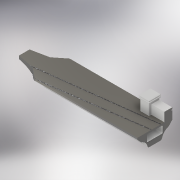
# Autodesk Inventor part: AC
Saved by Autodesk Inventor 2019 (Build 230136000, 136)
## iProperties
Created: 2020-08-10
Part Number: AC
Material: Generic
Document SubType Name: Modeling
Designer: Manoj
Density: 1 g/cm^3
Appearance: Default
Author: Manoj
Autodesk Inventor part; units mm, degrees
ref_plane "YZ Plane" through (0, 0, 0) normal (1, 0, 0) x (0, 1, 0)
ref_plane "XZ Plane" through (0, 0, 0) normal (0, 1, 0) x (-1, 0, 0)
ref_plane "XY Plane" through (0, 0, 0) normal (0, 0, 1) x (1, 0, 0)
sketch "Sketch1" plane through (0, 0, 0) normal (0, 1, 0) x (-1, 0, 0)
  line L0 (0, 0) -> (0, -10)
  line L1 (0, 0) -> (0, 10)
  line L2 (0, 0) -> (75, 0)
  line L3 (75, 0) -> (75, -3)
  line L4 (75, -3) -> (65.202, -5)
  line L5 (65.202, -5) -> (58.957, -10)
  line L6 (0, -10) -> (58.957, -10)
  line L7 (0, 0) -> (0, 10)
  line L8 (75, 0) -> (75, 3)
  line L9 (75, 3) -> (65.202, 5)
  line L10 (65.202, 5) -> (58.957, 10)
  line L11 (0, 10) -> (58.957, 10)
  point P0 (0, -5)
  dimension "d0" = 10
  dimension "d1" = 10
  dimension "d2" = 75
  dimension "d3" = 3
  dimension "d4" = 10
  dimension "d5" = 8
  constraints: 24 end point, 3 symmetric about line, 2 horizontal, 2 horizontal alignment, 2 vertical, 1 midpoint, 1 perpendicular
  measures "d0" distance of L0.start L0.end
  measures "d1" distance of L0.start L1.end
  measures "d2" distance of L0.start L2.end
  measures "d3" distance of L2.end L3.end
  measures "d4" distance of L3.end L4.end
  measures "d5" distance of L4.end L5.end
extrude "Extrusion1" add sketch "Sketch1" against normal blind 8
sketch "Sketch2" plane through (0, 0, 10) normal (1, 0, 0) x (0, 0, -1)
  line L0 (0, 0) -> (0, -8) projected
  line L1 (0, 0) -> (0, -3)
  line L2 (20, 0) -> (20, -8) projected
  line L3 (20, 0) -> (20, -3)
  line L4 (0, -8) -> (6, -8)
  line L5 (0, -8) -> (5, -8) projected
  line L6 (20, -8) -> (14, -8)
  line L7 (15, -8) -> (20, -8) projected
  arc A0 (6, -8) -> (0, -3) centre (0.4305, -8.5834) ccw
  line L8 (10, 0) -> (10, -8) construction
  line L9 (7, -8) -> (13, -8) construction
  arc A1 (20, -3) -> (14, -8) centre (19.5695, -8.5834) ccw
  line L10 (0, -3) -> (0, -8)
  line L11 (20, -3) -> (20, -8)
  dimension "d9" = 3
  dimension "d10" = 3
  dimension "d11" = 6
  dimension "d12" = 6
  dimension "d13" = 5.6
  dimension "d14" = 5.6
  constraints: 14 end point, 4 point on circle, 4 point on line, 2 centre point, 2 collinear, 1 midpoint
  measures "d9" distance of L0.start L1.end
  measures "d10" distance of L2.start L3.end
  measures "d11" distance of L0.end L4.end
  measures "d12" distance of L2.end L6.end
  measures "d13" radius of A0
  measures "d14" radius of A1
extrude "Extrusion2" cut sketch "Sketch2" against normal through all
sketch "Sketch3" plane through (0, 0, 0) normal (0, 0, 1) x (1, 0, 0)
  line L0 (-75, 0) -> (-75, -8) projected
  arc A0 (-58.9071, -7.8751) -> (-75, -1.8362) centre (-73.8044, -23.1121) ccw
  line L1 (-75, -1.8362) -> (-75, -12.4451)
  line L2 (-75, -12.4451) -> (-58.9071, -12.4451)
  line L3 (-58.9071, -12.4451) -> (-58.9071, -7.8751)
  point P0 (0, 0)
  constraints: 6 end point, 2 perpendicular, 2 point on circle, 1 centre point, 1 point on line, 1 vertical
extrude "Extrusion3" cut sketch "Sketch3" along normal through all both and the other way through all
fillet "Fillet1" radius 1 3 edges at (-58.9071, -8, 0) (-29.4536, -8, 4) (-29.4536, -8, -4)
sketch "Sketch4" plane through (0, 0, 0) normal (0, 1, 0) x (1, 0, 0)
  line L0 (-58.957, -10) -> (0, -10) projected
  line L1 (-58.957, -10) -> (0, -1.756)
  line L2 (-52.0795, -7.5) -> (0, 0)
  line L3 (-65.202, -5) -> (0, 3.1623)
  line L4 (-55.3465, -10) -> (0, -2.2608)
  line L5 (-66.7322, -4.6877) -> (0, 3.6662)
  line L6 (-75, -3) -> (-65.202, -5) projected
  line L7 (0, -10) -> (0, 10) projected
  line L8 (0, -2.2608) -> (0, -1.756)
  line L9 (-55.3465, -10) -> (-58.9488, -9.9988)
  line L10 (-66.7322, -4.6877) -> (-65.202, -5)
  line L11 (0, 3.1623) -> (0, 3.6662)
  dimension "d20" = 0.5
  dimension "d21" = 0.5
  constraints: 18 end point, 6 point on line, 3 collinear, 2 parallel
  measures "d20" distance between parallel lines of L1 L4
  measures "d21" distance between parallel lines of L3 L5
extrude "Extrusion4" add sketch "Sketch4" along normal blind 0.1 contours L1 L7 L4 L0 | L6 L5 L7 L3
sketch "Sketch5" plane through (0, 0, 0) normal (0, 1, 0) x (1, 0, 0)
  line L0 (0, 10) -> (-58.957, 10) projected
  line L1 (0, 10) -> (-7.5, 10)
  line L2 (-7.5, 10) -> (-7.5, 5.5)
  line L3 (-7.5, 5.5) -> (0, 5.5)
  line L4 (0, 5.5) -> (0, 10)
  point P0 (0, 0)
  dimension "d24" = 7.5
  dimension "d25" = 4.5
  constraints: 8 end point, 2 parallel, 1 horizontal, 1 perpendicular
  measures "d24" distance of L3.end L2.end
  measures "d25" distance of L2.end L1.end
extrude "Extrusion5" add sketch "Sketch5" along normal blind 5.2
sketch "Sketch6" plane through (0, 0, 0) normal (0, 1, 0) x (1, 0, 0)
  line L0 (0, 10) -> (-7.5, 10) projected
  line L1 (-7.5, 10) -> (-12.5, 10)
  line L2 (-12.5, 10) -> (-12.5, 4.2)
  line L3 (-12.5, 4.2) -> (-7.5, 4.2)
  line L4 (-7.5, 4.2) -> (-7.5, 10)
  point P0 (0, 0)
  dimension "d28" = 5
  dimension "d29" = 5.8
  constraints: 8 end point, 2 parallel, 1 horizontal, 1 perpendicular
  measures "d28" distance of L3.end L2.end
  measures "d29" distance of L2.end L1.end
extrude "Extrusion6" add sketch "Sketch6" along normal blind 6.5
sketch "Sketch7" plane through (0, -3, 10) normal (1, 0, 0) x (0, 0, -1)
  arc A0 (13.1623, -5) -> (14.1331, -4.2399) centre (13.1623, -4) ccw projected
  arc A1 (20, 0) -> (14.1331, -4.2399) centre (19.5695, -5.5834) ccw projected
  line L0 (20, 0) -> (20, 8.2) projected
  line L1 (15.5, 8.2) -> (20, 8.2) projected
  line L2 (15.5, 3) -> (15.5, 8.2) projected
  line L3 (13.6662, 3) -> (15.5, 3) projected
  line L4 (13.6662, 3) -> (13.6662, 3.1) projected
  line L5 (13.1623, 3.1) -> (13.6662, 3.1) projected
  line L6 (13.1623, 3) -> (13.1623, 3.1) projected
  line L7 (8.244, 3) -> (13.1623, 3) projected
  line L8 (8.244, 3) -> (8.244, 3.1) projected
  line L9 (7.7392, 3.1) -> (8.244, 3.1) projected
  line L10 (7.7392, 3) -> (7.7392, 3.1) projected
  line L11 (0, 3) -> (7.7392, 3) projected
  line L12 (0, 3) -> (0, 0) projected
  arc A2 (5.8669, -4.2399) -> (0, 0) centre (0.4305, -5.5834) ccw projected
  arc A3 (5.8669, -4.2399) -> (6.8377, -5) centre (6.8377, -4) ccw projected
  line L13 (13.1623, -5) -> (6.8377, -5) projected
  line L14 (13.1623, -5) -> (6.8377, -5) projected
  arc A4 (5.8669, -4.2399) -> (6.8377, -5) centre (6.8377, -4) ccw projected
  arc A5 (5.8669, -4.2399) -> (0, 0) centre (0.4305, -5.5834) ccw projected
  line L15 (0, 0) -> (0, 3) projected
  line L16 (0, 3) -> (7.7392, 3) projected
  line L17 (7.7392, 3) -> (7.7392, 3.1) projected
  line L18 (8.244, 3.1) -> (8.244, 3) projected
  line L19 (8.244, 3) -> (13.1623, 3) projected
  line L20 (13.1623, 3) -> (13.1623, 3.1) projected
  line L21 (13.1623, 3.1) -> (13.6662, 3.1) projected
  line L22 (13.6662, 3) -> (15.5, 3) projected
  line L23 (15.5, 3) -> (15.5, 8.2) projected
  line L24 (15.5, 8.2) -> (20, 8.2) projected
  line L25 (20, 8.2) -> (20, 0) projected
  arc A6 (20, 0) -> (14.1331, -4.2399) centre (19.5695, -5.5834) ccw projected
  arc A7 (13.1623, -5) -> (14.1331, -4.2399) centre (13.1623, -4) ccw projected
  line L26 (20, 3) -> (15, 3) projected
  line L27 (15.5, 3) -> (20, 3)
  line L28 (15.5, 3) -> (15.5, 8.2) projected
  line L29 (0, 3) -> (7.7392, 3) projected
  line L30 (8.244, 3) -> (13.1623, 3) projected
  line L31 (6, 2) -> (14, 2)
  line L32 (14.5, 1.5) -> (14.5, -1.5)
  line L33 (14, -2) -> (6, -2)
  line L34 (5.5, -1.5) -> (5.5, 1.5)
  arc A8 (5.5, -1.5) -> (6, -2) centre (6, -1.5) ccw
  arc A9 (14.5, 1.5) -> (14, 2) centre (14, 1.5) ccw
  arc A10 (6, 2) -> (5.5, 1.5) centre (6, 1.5) ccw
  arc A11 (14, -2) -> (14.5, -1.5) centre (14, -1.5) ccw
  line L35 (7.7392, 3.1) -> (8.244, 3.1) projected
  line L36 (13.6662, 3.1) -> (13.6662, 3) projected
  point P0 (10, 3)
  point P1 (10, 2)
  point P2 (14.5, 0)
  dimension "d32" = 0.5
  dimension "d33" = 0.5
  dimension "d36" = 8
  dimension "d37" = 3
  constraints: 10 end point, 8 point on circle, 8 tangent, 4 centre point, 2 equal radius, 2 midpoint, 2 parallel, 1 collinear, 1 horizontal, 1 horizontal alignment, 1 perpendicular, 1 vertical alignment
  measures "d32" radius of A8
  measures "d33" radius of A9
  measures "d36" distance of L31.start L31.end
  measures "d37" distance of L34.start L34.end
extrude "Extrusion7" cut sketch "Sketch7" against normal blind 50 contours L31 A9 L32 A11 L33 A8 L34 A10
chamfer "Chamfer1" distance 2 angle 45 2 edges at (-29.4785, -3, -10) (-29.4785, -3, 10)
sketch "Sketch8" plane through (0, 6.5, 0) normal (0, 1, 0) x (1, 0, 0)
  line L0 (-7.5, 10) -> (-12.5, 10) projected
  line L1 (-12.5, 10) -> (-12.5, 4.2) projected
  line L2 (-12.5, 4.2) -> (-7.5, 4.2) projected
  line L3 (-7.5, 4.2) -> (-7.5, 10) projected
  line L4 (-13, 3.7) -> (-13, 10.5)
  line L5 (-13, 10.5) -> (-7, 10.5)
  line L6 (-7, 10.5) -> (-7, 3.7)
  line L7 (-7, 3.7) -> (-13, 3.7)
  point P0 (0, 0)
  dimension "d41" = 0.5
  constraints: 8 end point, 3 other
  measures "d41" distance between parallel lines of L1 L4
extrude "Extrusion8" add sketch "Sketch8" along normal blind 0.4 contours L3 L2 L1 L0 | L4 L5 L6 L7
sketch "Sketch9" plane through (0, 6.9, 0) normal (0, 1, 0) x (1, 0, 0)
  line L0 (-13, 10.5) -> (-13, 3.7) projected
  line L1 (-13, 3.7) -> (-7, 3.7) projected
  line L2 (-7, 3.7) -> (-7, 10.5) projected
  line L3 (-7, 10.5) -> (-13, 10.5) projected
  line L4 (-12.6, 4.1) -> (-12.6, 10.1)
  line L5 (-12.6, 10.1) -> (-7.4, 10.1)
  line L6 (-7.4, 10.1) -> (-7.4, 4.1)
  line L7 (-7.4, 4.1) -> (-12.6, 4.1)
  point P0 (0, 0)
  dimension "d44" = 0.4
  constraints: 8 end point, 3 other
  measures "d44" distance between parallel lines of L0 L4
extrude "Extrusion9" add sketch "Sketch9" along normal blind 0.6 contours L4 L5 L6 L7
sketch "Sketch10" plane through (0, 7.5, 0) normal (0, 1, 0) x (1, 0, 0)
  line L0 (-12.6, 10.1) -> (-12.6, 4.1) projected
  line L1 (-12.6, 4.1) -> (-7.4, 4.1) projected
  line L2 (-7.4, 4.1) -> (-7.4, 10.1) projected
  line L3 (-7.4, 10.1) -> (-12.6, 10.1) projected
  line L4 (-13, 3.7) -> (-13, 10.5)
  line L5 (-13, 10.5) -> (-7, 10.5)
  line L6 (-7, 10.5) -> (-7, 3.7)
  line L7 (-7, 3.7) -> (-13, 3.7)
  point P0 (0, 0)
  dimension "d47" = 0.4
  constraints: 8 end point, 3 other
  measures "d47" distance between parallel lines of L0 L4
extrude "Extrusion10" add sketch "Sketch10" along normal blind 0.4 contours L3 L2 L1 L0 | L4 L5 L6 L7
sketch "Sketch11" plane through (0, -8, 3.1623) normal (1, 0, 0) x (0, 0, -1)
  line L0 (8.6389, 12.2685) -> (9.0577, 12.2685)
  line L1 (9.0577, 12.2685) -> (9.0577, 11.7208)
  line L2 (9.0577, 11.7208) -> (8.6389, 11.7208)
  line L3 (8.6389, 11.7208) -> (8.6389, 12.2685)
  line L4 (13.1623, 7) -> (13.1623, 13.2) projected
  line L5 (13.1623, 12.2685) -> (12.8268, 12.2685)
  line L6 (12.8268, 12.2685) -> (12.8268, 11.7208)
  line L7 (12.8268, 11.7208) -> (13.1623, 11.7208)
  line L8 (13.1623, 11.7208) -> (13.1623, 12.2685)
  point P0 (3.1623, 8)
  constraints: 16 end point, 4 parallel, 3 point on line, 2 horizontal, 2 perpendicular
extrude "Extrusion11" cut sketch "Sketch11" against normal blind 21.75 contours L7 L6 L5 L4
sketch "Sketch12" plane through (0, 0, 0) normal (0, 0, 1) x (1, 0, 0)
  line L0 (-13.0285, -3.1035) -> (-47.3972, -3.1035)
  line L1 (-47.3972, -3.1035) -> (-47.3972, -5)
  line L2 (-47.3972, -5) -> (-13.0285, -5)
  line L3 (-13.0285, -5) -> (-13.0285, -3.1035)
  line L4 (0, -5) -> (-50, -5) projected
  point P0 (0, 0)
  constraints: 8 end point, 2 parallel, 1 collinear, 1 horizontal, 1 perpendicular
extrude "Extrusion12" cut sketch "Sketch12" against normal blind 21.75
body "Solid1"
